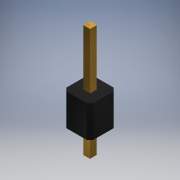
# Autodesk Inventor part: CON-PIN-L11
Saved by Autodesk Inventor 2018.3 (Build 223284000, 284)
## iProperties
Created: 2020-10-22
Part Number: CON-PIN-L11
Material: Genérico
Document SubType Name: Modeling
Designer: laguerre
Density: 8.47 g/cm^3
Appearance: Valor por defecto
Author: laguerre
Autodesk Inventor part; units mm, degrees
ref_plane "YZ Plane" through (0, 0, 0) normal (1, 0, 0) x (0, 1, 0)
ref_plane "XZ Plane" through (0, 0, 0) normal (0, 1, 0) x (-1, 0, 0)
ref_plane "XY Plane" through (0, 0, 0) normal (0, 0, 1) x (1, 0, 0)
sketch "Boceto39" plane through (0, 0, 0) normal (0, 0, 1) x (1, 0, 0)
  line L0 (-0.32, 5.46) -> (0.32, 5.46)
  line L1 (0.32, 5.46) -> (0.32, 0)
  line L2 (0.32, 0) -> (-0.32, 0)
  line L3 (-0.32, 0) -> (-0.32, 5.46)
  line L4 (0.32, 0) -> (-0.32, 0)
  line L5 (-0.32, 0) -> (-0.32, -5.54)
  line L6 (-0.32, -5.54) -> (0.32, -5.54)
  line L7 (0.32, -5.54) -> (0.32, 0)
  point P0 (0, 0)
  point P1 (0, 5.46)
  point P2 (0, 0)
  dimension "d373" = 0.64
  dimension "d375" = 5.54
  dimension "d392" = 11
  dimension "d393" = 5.46
  constraints: 16 end point, 4 parallel, 2 horizontal, 2 midpoint, 2 perpendicular, 1 coincident, 1 point on line, 1 vertical alignment
  measures "d373" distance between parallel lines of L1 L3
  measures "d375" distance from line of L6 point (0, 0)
  measures "d392" distance from line of point (0, 5.46) L6
  measures "d393" distance from line of point (0, 0) L0
extrude "Extrusión13" add sketch "Boceto39" along normal mid plane 0.64
chamfer "Chaflán5" distance 0.2 angle 45 8 edges at (0.32, 5.46, 0) (0, 5.46, 0.32) (-0.32, 5.46, 0) (0, 5.46, -0.32) (-0.32, -5.54, 0) (0, -5.54, 0.32) (0.32, -5.54, 0) (0, -5.54, -0.32)
sketch "Boceto40" plane through (0, 0, 0) normal (0, 1, 0) x (-1, 0, 0)
  line L0 (-0.97, -1.27) -> (0.97, -1.27)
  line L1 (1.27, -0.97) -> (1.27, 0.97)
  line L2 (0.97, 1.27) -> (-0.97, 1.27)
  line L3 (-1.27, 0.97) -> (-1.27, -0.97)
  line L4 (-1.27, -0.97) -> (-0.97, -1.27)
  line L5 (1.27, -0.97) -> (0.97, -1.27)
  line L6 (0.97, 1.27) -> (1.27, 0.97)
  line L7 (-0.97, 1.27) -> (-1.27, 0.97)
  point P0 (0, 0)
  point P1 (-1.27, -1.27)
  point P2 (1.27, 1.27)
  point P3 (1.27, -1.27)
  point P4 (-1.27, 1.27)
  point P5 (0, -1.27)
  point P6 (-1.27, 0)
  dimension "d381" = 2.54
  dimension "d382" = 0.3
  dimension "d383" = 0.3
  dimension "d384" = 0.3
  dimension "d385" = 0.3
  dimension "d386" = 0.3
  dimension "d387" = 0.3
  dimension "d388" = 0.3
  dimension "d389" = 0.3
  constraints: 16 end point, 8 point on line, 2 midpoint, 2 parallel, 2 perpendicular, 1 horizontal, 1 horizontal alignment, 1 vertical alignment
  measures "d381" distance of point (-1.27, -1.27) point (1.27, -1.27)
  measures "d382" distance of L3.end point (-1.27, -1.27)
  measures "d383" distance of L0.start point (-1.27, -1.27)
  measures "d384" distance of L1.start point (1.27, -1.27)
  measures "d385" distance of L0.end point (1.27, -1.27)
  measures "d386" distance of L2.start point (1.27, 1.27)
  measures "d387" distance of L1.end point (1.27, 1.27)
  measures "d388" distance of L2.end point (-1.27, 1.27)
  measures "d389" distance of L3.start point (-1.27, 1.27)
extrude "Extrusión14" add sketch "Boceto40" against normal blind 3
